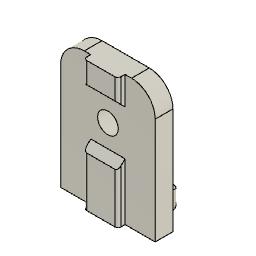
Z Rail Stop (Autodesk Fusion 360 design; units mm, degrees)
Autodesk Fusion 360 part; units mm, degrees
note: some values were not read from the file. Set by a fixed rule: which sketch regions a step uses.
sketch "Sketch1" plane through (0, 0, 0) normal (0, 1, 0) x (1, 0, 0)
  line L0 (8, 11) -> (-8, 11)
  line L1 (-8, 11) -> (-8, -11)
  line L2 (-8, -11) -> (8, -11)
  line L3 (8, -11) -> (8, 11)
  line L4 (8, 11) -> (-8, -11) construction
  line L5 (-8, 11) -> (8, -11) construction
  dimension "d1" = 16
  dimension "d3" = 22
  constraint horizontal L0
  constraint perpendicular L0 L1
  constraint parallel L0 L2
  constraint parallel L1 L3
  constraint coincident L4 origin
  constraint coincident L5 origin
  measures "d1" distance of L1.end L2.end
  measures "d3" distance of L0.start L2.end
extrude "Extrude1" add sketch "Sketch1" along normal blind 3
sketch "Sketch2" plane through (0, 0, 11) normal (0, 0, 1) x (-1, 0, 0)
  line L0 (8, 0) -> (-8, 0)
  line L1 (-8, 0) -> (-8, -3)
  line L2 (-8, -3) -> (8, -3)
  line L3 (8, -3) -> (8, 0)
  line L4 (2.9, 0) -> (-2.9, 0)
  line L5 (-2.9, 0) -> (-2.9, 1.2)
  line L6 (-2.9, 1.2) -> (2.9, 1.2)
  line L7 (2.9, 1.2) -> (2.9, 0)
  dimension "d6" = 5.8
  dimension "d7" = 1.2
  constraint horizontal L4
  constraint vertical L5
  constraint horizontal L6
  constraint vertical L7
  constraint coincident L0 L4.start
  constraint midpoint origin L4
  measures "d6" distance of L4.start L4.end
  measures "d7" distance of L4.end L5.end
extrude "Extrude2" add sketch "Sketch2" against normal up to surface (22 mm away) contours L0 L4 L5 L6 L7
fillet "Fillet1" radius 0.5 2 edges at (2.9, -1.2, 0) (-2.9, -1.2, 0)
sketch "Sketch4" plane through (-8, 0, 0) normal (-1, 0, 0) x (0, -1, 0)
  line L0 (0, -11) -> (0, 11)
  line L1 (0, 11) -> (-3, 11)
  line L2 (-3, 11) -> (-3, -11)
  line L3 (-3, -11) -> (0, -11)
  line L4 (-3, -11) -> (-8, -11)
  line L5 (-8, -11) -> (-8, -9)
  line L6 (-8, -9) -> (-3, -6.1132)
  dimension "d15" = 5
  dimension "d22" = 2
  dimension "d23" = 120
  constraint coincident L2.end L3.start
  constraint perpendicular L2 L4
  constraint perpendicular L4 L5
  constraint coincident L2 L6.end
  measures "d15" distance of L2.end L4.end
  measures "d22" distance of L4.end L5.end
  measures "d23" angle of L5 L6
extrude "Extrude4" add sketch "Sketch4" against normal up to surface (16 mm away) contours L2 L4 L5 L6
sketch "Sketch5" plane through (0, 0, -11) normal (0, 0, -1) x (1, 0, 0)
  arc A0 (-2.4, 1.2) -> (-2.9, 0.7) centre (-2.4, 0.7) ccw
  line L0 (-2.9, 0.7) -> (-2.9, 0)
  line L1 (-2.9, 0) -> (-8, 0)
  line L2 (-8, 0) -> (-8, -8)
  line L3 (8, -8) -> (8, 0)
  line L4 (8, 0) -> (2.9, 0)
  line L5 (2.9, 0) -> (2.9, 0.7)
  arc A1 (2.9, 0.7) -> (2.4, 1.2) centre (2.4, 0.7) ccw
  line L6 (2.4, 1.2) -> (-2.4, 1.2)
  line L7 (-8, -8) -> (8, -8)
  line L8 (-8, -3) -> (8, -3)
  line L9 (-5, -8) -> (5, -8)
  line L10 (5, -8) -> (5, -3)
  line L11 (5, -3) -> (-5, -3)
  line L12 (-5, -3) -> (-5, -8)
  dimension "d30" = 10
  constraint horizontal L9
  constraint vertical L10
  constraint horizontal L11
  constraint vertical L12
  constraint coincident L8 L10.end
  constraint coincident L7 L9.start
  constraint midpoint L7 L9
  measures "d30" distance of L9.start L9.end
extrude "Extrude5" cut sketch "Sketch5" against normal through all contours L2 L7 L8 L12 | L3 L7 L8 L10
sketch "Sketch6" plane through (0, 3, 0) normal (0, 1, 0) x (-1, 0, 0)
  line L0 (-5, -6.1132) -> (5, -6.1132)
  line L1 (8, -11) -> (8, 11)
  line L2 (8, 11) -> (-8, 11)
  line L3 (-8, 11) -> (-8, -11)
  circle A0 centre (0, 2.4434) radius 1.75
  line L4 (5, -6.1132) -> (5, -11)
  line L5 (5, -11) -> (8, -11)
  line L6 (-8, -11) -> (-5, -11)
  line L7 (-5, -11) -> (-5, -6.1132)
  line L8 (0, -6.1132) -> (0, 11)
  dimension "d24" = 3.5
  constraint midpoint L0 L8.start
  constraint midpoint L2 L8.end
  constraint midpoint A0.centre L8
  measures "d24" diameter of A0
extrude "Extrude6" cut sketch "Sketch6" against normal through all contours A0 L8 | A0 L8
sketch "Sketch7" plane through (0, 0, 0) normal (0, -1, 0) x (1, 0, 0)
  line L0 (-2.9, -11) -> (-2.9, 11) construction
  line L1 (-2.9, 11) -> (-8, 11)
  line L2 (-8, 11) -> (-8, -11)
  line L3 (-8, -11) -> (-2.9, -11)
  line L4 (-8, 7.4434) -> (8, 7.4434)
  line L5 (8, 7.4434) -> (8, -2.5566)
  line L6 (8, -2.5566) -> (-8, -2.5566)
  line L7 (-8, -2.5566) -> (-8, 7.4434)
  line L8 (2.9, 11) -> (2.9, -11) construction
  line L9 (2.9, -11) -> (8, -11)
  line L10 (8, -11) -> (8, 11)
  line L11 (8, 11) -> (2.9, 11)
  line L12 (-8, 2.4434) -> (8, 2.4434)
  circle A0 centre (0, 2.4434) radius 1.75
  dimension "d26" = 10
  constraint horizontal L4
  constraint vertical L5
  constraint horizontal L6
  constraint vertical L7
  constraint coincident L2 L4.start
  constraint coincident L5.end L10
  constraint midpoint L7 L12.start
  constraint midpoint L5 L12.end
  constraint coincident L12 A0.centre
  measures "d26" distance of L4.start L6.end
extrude "Extrude7" cut sketch "Sketch7" along normal through all contours L2 L4 L5 L7 L10 L12 A0 | L2 L5 L6 L7 L10 L12 A0
fillet "Fillet2" radius 4 2 edges at (-8, 1.5, 11) (8, 1.5, 11)
fillet "Fillet3" radius 2.5 4 edges at (-5, 8, -10) (5, 8, -10) (-5, 3, -8.5566) (5, 3, -8.5566)
draft "Draft1" angle 45 neutral plane through (2.9, -1.2, 11) pull (0, -1, 0) 2 faces at (0.8, -0.4, 7.4434) (0.8, -0.4, -2.5566)
